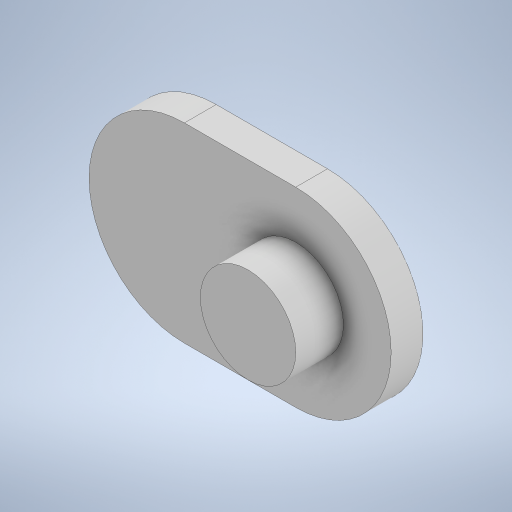
# Autodesk Inventor part: wrist_gear_spacer
Saved by Autodesk Inventor 2024.1 (Build 281209000, 209)
## iProperties
Created: 2025-03-02
Part Number: wrist_gear_spacer
Material: 一般
Document SubType Name: Modeling
Designer: hibik
Density: 1 g/cm^3
Appearance: 既定
Author: hibik
Autodesk Inventor part; units mm, degrees
ref_plane "YZ Plane" through (0, 0, 0) normal (1, 0, 0) x (0, 1, 0)
ref_plane "XZ Plane" through (0, 0, 0) normal (0, 1, 0) x (-1, 0, 0)
ref_plane "XY Plane" through (0, 0, 0) normal (0, 0, 1) x (1, 0, 0)
sketch "スケッチ1" plane through (0, 0, 0) normal (0, 0, 1) x (1, 0, 0)
  circle A0 centre (0, 0) radius 17.5 construction
  circle A1 centre (-7, 0) radius 10.5 construction
  circle A2 centre (-7, 0) radius 6
  circle A3 centre (0, 0) radius 6
  line L0 (-7, 6) -> (0, 6)
  line L1 (0, 6) -> (0, -6) construction
  line L2 (0, -6) -> (-7, -6)
  line L3 (-7, -6) -> (-7, 6) construction
  dimension "d2" = 12
  dimension "d3" = 12
  dimension "d0" = 35
  dimension "d1" = 21
  constraints: 8 end point, 3 coincident, 3 horizontal, 2 centre point, 2 parallel, 1 horizontal alignment, 1 perpendicular, 1 tangent, 6 other
  measures "d0" diameter of A0
  measures "d1" diameter of A1
extrude "押し出し1" add sketch "スケッチ1" along normal blind 2
sketch "スケッチ2" plane through (0, 0, 2) normal (0, 0, 1) x (1, 0, 0)
  circle A0 centre (0, 0) radius 3
  dimension "d6" = 6
  constraints: 1 centre point, 1 coincident
  measures "d6" diameter of A0
extrude "押し出し2" add sketch "スケッチ2" along normal blind 3
sketch "スケッチ3" plane through (0, 0, 0) normal (0, 0, -1) x (-1, 0, 0)
  arc A0 (7, -6) -> (7, 6) centre (7, 0) ccw projected
  circle A1 centre (7, 0) radius 3
  point P0 (0, 0)
  dimension "d9" = 6
  constraints: 1 centre point, 1 coincident
  measures "d9" diameter of A1
extrude "押し出し3" add sketch "スケッチ3" along normal blind 3
